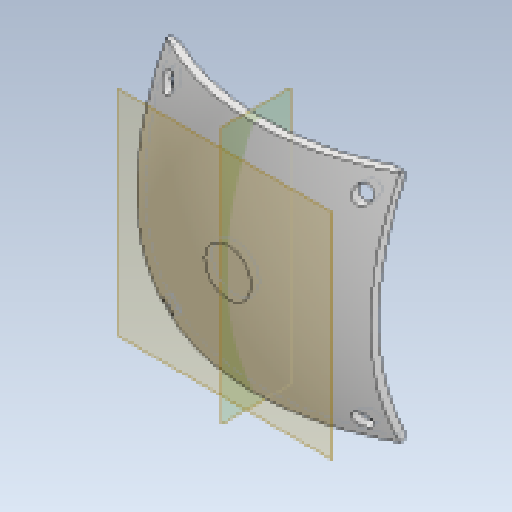
# Autodesk Inventor part: sling
Saved by Autodesk Inventor 2023 (Build 270158030, 158C)
## iProperties
Created: 2024-12-21
Part Number: sling
Material: Generic
Document SubType Name: Modeling
Designer: Imogen Heard
Density: 1 g/cm^3
Appearance: Default
Author: Imogen Heard
Autodesk Inventor part; units mm, degrees
ref_plane "YZ Plane" through (0, 0, 0) normal (1, 0, 0) x (0, 1, 0)
ref_plane "XZ Plane" through (0, 0, 0) normal (0, 1, 0) x (-1, 0, 0)
ref_plane "XY Plane" through (0, 0, 0) normal (0, 0, 1) x (1, 0, 0)
ref_plane "Work Plane1" through (0, 75, 0) normal (0, 0, 1) x (-1, 0, 0)
sketch "Sketch1" plane through (0, 75, 0) normal (0, 0, 1) x (-1, 0, 0)
  line L0 (-15, 15) -> (15, 15)
  line L1 (15, 15) -> (15, -15)
  line L2 (15, -15) -> (-15, -15)
  line L3 (-15, -15) -> (-15, 15)
  spline S0 degree 3 poles (-65.846498, 1.129483) (-66.023415, 1.035237) (-66.184792, 0.911656) (-66.420387, 0.634892) (-66.503383, 0.492913) (-66.593364, 0.215406) (-66.611641, 0.088428) (-66.601873, -0.174872) (-66.571521, -0.306599) (-66.462409, -0.56455) (-66.381946, -0.686116) (-66.166388, -0.923449) (-66.024815, -1.031201) (-65.673495, -1.225315) (-65.455304, -1.297569) (-64.958992, -1.379475) (-64.675012, -1.371901) (-64.167394, -1.258191) (-63.938061, -1.163548) (-63.586794, -0.921291) (-63.452663, -0.791861) (-63.263361, -0.51093) (-63.200982, -0.368705) (-63.1464, -0.102069) (-63.141607, 0.015187) (-63.173205, 0.271637) (-63.217391, 0.405723) (-63.354598, 0.661931) (-63.448656, 0.779762) (-63.694371, 1.008117) (-63.853336, 1.109294) (-64.240838, 1.282805) (-64.47753, 1.339681) (-64.90734, 1.371511) (-65.101317, 1.3605) (-65.483475, 1.286641) (-65.67267, 1.222084) (-65.846498, 1.129483) knots 0 0 0 0 0.06013616 0.06013616 0.10939739 0.10939739 0.14811685 0.14811685 0.18887866 0.18887866 0.23253514 0.23253514 0.2853526 0.2853526 0.35301463 0.35301463 0.4359349 0.4359349 0.508779 0.508779 0.56418283 0.56418283 0.61088227 0.61088227 0.64633433 0.64633433 0.68887198 0.68887198 0.73395435 0.73395435 0.78981498 0.78981498 0.8613873 0.8613873 0.91886474 0.91886474 0.97795104 0.97795104 0.97795104 0.97795104
  line L4 (50, 27.5) -> (-50, 27.5)
  line L5 (-50, -27.5) -> (50, -27.5)
  point P0 (0, 75)
  point P1 (-65.846498, 1.129483)
  dimension "d0" = 30
  dimension "d1" = 30
  dimension "d2" = 15
  dimension "d3" = 12.5
  dimension "d4" = 12.5
  constraints: 8 end point, 2 parallel, 1 horizontal, 1 perpendicular
  measures "d0" distance between parallel lines of L1 L3
  measures "d1" distance between parallel lines of L2 L0
  measures "d2" distance from line of L3 point (0, 75)
  measures "d3" distance between parallel lines of L0 L4
  measures "d4" distance between parallel lines of L5 L2
sketch "Sketch1 outline for Extrusion1" plane through (0, 75, 0) normal (0, 0, 1) x (-1, 0, 0)
  line L0 (-15, 15) -> (-15, -15)
  line L1 (15, 15) -> (-15, 15)
  line L2 (15, -15) -> (15, 15)
  line L3 (-15, -15) -> (15, -15)
extrude "Extrusion1" add sketch "Sketch1 outline for Extrusion1" against normal blind 8
ref_plane "Work Plane2" through (0, 60, 0) normal (-1, 0, 0) x (0, 0, 1)
sketch "Sketch2" plane through (0, 60, 0) normal (-1, 0, 0) x (0, 0, 1)
  line L0 (0, 30) -> (0, 0)
  line L1 (0, 30) -> (-8, 30)
  line L2 (-8, 0) -> (-8, 30)
  line L3 (0, 0) -> (-8, 0)
  line L4 (-15.43696, 15) -> (9.946086, 15)
  line L5 (0, 0) -> (-8, 0)
  line L6 (0, 0) -> (-8, 0)
  line L7 (0, 30) -> (-8, 30)
  line L8 (-6, 0) -> (-8, 0)
  line L9 (-6, 30) -> (-8, 30)
  line L10 (0, 0) -> (-8, 0)
  line L11 (-8, 30) -> (0, 30)
  line L12 (0, 0) -> (0, 30)
  line L13 (0, 0) -> (-8, 0)
  line L14 (-8, 0) -> (-8, -11)
  line L15 (-8, -11) -> (0, -11)
  line L16 (0, -11) -> (0, 0)
  line L17 (-8, 30) -> (0, 30)
  line L18 (0, 30) -> (0, 41)
  line L19 (0, 41) -> (-8, 41)
  line L20 (-8, 41) -> (-8, 30)
  line L21 (-1.4, 15) -> (-0.4, 15)
  line L22 (-0.4, 15) -> (-0.4, 12)
  line L23 (-0.4, 12) -> (-1.4, 12)
  line L24 (-1.4, 12) -> (-1.4, 15)
  line L25 (0, 30) -> (0, 0)
  arc A0 (-13, -11) -> (-1.4, 12) centre (-37.215674, 15.63834) ccw
  line L26 (-13, -11) -> (-12, -11)
  arc A1 (-12, -11) -> (-0.4, 12) centre (-35.257502, 15.155088) ccw
  point P0 (0, -60)
  point P1 (-4, 0)
  point P2 (-8, 15)
  point P3 (0, 15)
  point P4 (-6, 0)
  point P5 (0, 15)
  point P6 (0, 15)
  point P7 (0, 15)
  point P8 (0, 15)
  point P9 (-8, 0)
  point P10 (-8, -6.800062)
  point P11 (-8, -5.396023)
  dimension "d9" = 15
  dimension "d19" = 15
  dimension "d20" = 11
  dimension "d21" = 11
  dimension "d22" = 4
  dimension "d31" = 1
  dimension "d32" = 0.4
  dimension "d33" = 1
  dimension "d34" = 3
  dimension "d35" = 35
  dimension "d36" = 36
  constraints: 36 end point, 7 horizontal, 6 parallel, 5 horizontal alignment, 4 coincident, 4 midpoint, 4 point on circle, 3 perpendicular, 3 point on line, 3 vertical alignment, 2 centre point, 2 collinear
  measures "d9" distance between parallel lines of L4 L1
  measures "d19" distance between parallel lines of L3 L4
  measures "d20" distance between parallel lines of L15 L3
  measures "d21" distance between parallel lines of L1 L19
  measures "d22" horizontal distance of L26.end L2.start
  measures "d31" distance between parallel lines of L24 L22
  measures "d32" distance from line of point (0, 15) L22
  measures "d33" distance of L26.start L26.end
  measures "d34" distance from line of point (0, 15) L23
  measures "d35" radius of A1
  measures "d36" radius of A0
sketch "Sketch2 outline for Revolution1" plane through (0, 60, 0) normal (-1, 0, 0) x (0, 0, 1)
  arc A0 (-0.4, 12) -> (-8, -6.800062) centre (-35.257502, 15.155088) cw
  line L0 (-8, -6.800062) -> (-8, -11)
  line L1 (-8, -11) -> (0, -11)
  line L2 (0, -11) -> (0, 15)
  line L3 (0, 15) -> (-0.4, 15)
  line L4 (-0.4, 15) -> (-0.4, 12)
  arc A1 (-8, -5.396023) -> (-1.4, 12) centre (-37.215674, 15.63834) ccw
  line L5 (-1.4, 12) -> (-1.4, 15)
  line L6 (-1.4, 15) -> (-8, 15)
  line L7 (-8, 15) -> (-8, -5.396023)
revolve "Revolution1" cut sketch "Sketch2 outline for Revolution1" angle 360 about axis through (0, 75, -15.43696) along (0, 0, 1)
sketch "Sketch3" plane through (0, 75, -8) normal (0, 0, -1) x (-1, 0, 0)
  circle A0 centre (-12.5, -12.5) radius 1
  line L0 (-15, 15) -> (-15, -15) projected
  line L1 (-15, -15) -> (15, -15) projected
  circle A1 centre (12.5, -12.5) radius 1
  circle A2 centre (-12.5, 12.5) radius 1
  circle A3 centre (12.5, 12.5) radius 1
  line L2 (15, -15) -> (15, 15) projected
  line L3 (15, 15) -> (-15, 15) projected
  point P0 (0, -75)
  point P1 (-15, -13.772809)
  point P2 (-13.772809, -15)
  point P3 (15, 13.772809)
  point P4 (13.772809, 15)
  dimension "d24" = 2
  dimension "d25" = 2.5
  dimension "d26" = 2.5
  dimension "d27" = 2.5
  dimension "d28" = 2.5
  constraints: 4 centre point, 3 equal radius, 2 horizontal alignment, 2 vertical alignment
  measures "d24" diameter of A0
  measures "d25" distance from line of L0 A0.centre
  measures "d26" distance from line of L1 A0.centre
  measures "d27" distance from line of L2 A3.centre
  measures "d28" distance from line of L3 A3.centre
sketch "Sketch3 outline for Extrusion2" plane through (0, 75, -8) normal (0, 0, -1) x (-1, 0, 0)
  circle A0 centre (12.5, -12.5) radius 1
  circle A1 centre (12.5, 12.5) radius 1
  circle A2 centre (-12.5, 12.5) radius 1
  circle A3 centre (-12.5, -12.5) radius 1
extrude "Extrusion2" cut sketch "Sketch3 outline for Extrusion2" against normal through all
equation "\"d1\" = d0"
equation "\"d25\" = d28"
equation "\"d26\" = d27"
